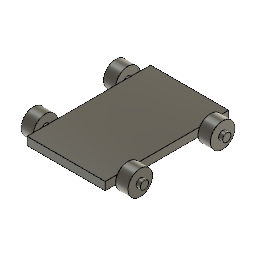
Semana3_DesafioExtra v1 (Autodesk Fusion 360 design; units mm, degrees)
Autodesk Fusion 360 part; units mm, degrees
sketch "Sketch2" plane through (0, 0, 0) normal (1, 0, 0) x (0, 1, 0)
  circle A0 centre (-50, 0) radius 15
  circle A1 centre (50, 0) radius 15
  dimension "d3" = 30
  dimension "d4" = 30
  dimension "d5" = 50
  dimension "d6" = 50
  constraint collinear origin A0.centre A1.centre
  measures "d3" diameter of A0
  measures "d4" diameter of A1
  measures "d5" distance of origin A0.centre
  measures "d6" distance of origin A1.centre
extrude "Extrude2" add sketch "Sketch2" along normal blind 15 makes body 1 at (10, 64.9255, -1.4935) makes body 2 at (10, -35.0745, -1.4935)
ref_plane "WorkPlane1" through (-100, 0, 0) normal (1, 0, 0) x (0, 1, 0)
sketch "Sketch3" plane through (-100, 0, 0) normal (1, 0, 0) x (0, 1, 0)
  circle A0 centre (50, 0) radius 15
  circle A1 centre (-50, 0) radius 15
  circle A2 centre (50, 0) radius 15
  circle A3 centre (-50, 0) radius 15
  dimension "d10" = 30
  dimension "d11" = 30
  constraint concentric A0 A2
  constraint concentric A1 A3
  measures "d10" diameter of A0
  measures "d11" diameter of A1
extrude "Extrude3" add sketch "Sketch3" against normal blind 15 separate body makes body 3 at (-110, 64.9255, -1.4935) makes body 4 at (-110, -35.0745, -1.4935)
sketch "Sketch4" plane through (15, 0, 0) normal (1, 0, 0) x (0, 1, 0)
  circle A0 centre (50, 0) radius 15
  circle A1 centre (50, 0) radius 5
  circle A2 centre (-50, 0) radius 5
  circle A3 centre (-50, 0) radius 15
  dimension "d14" = 10
  dimension "d15" = 10
  constraint concentric A0 A1
  constraint concentric A2 A3
  measures "d14" diameter of A1
  measures "d15" diameter of A2
extrude "Extrude4" add sketch "Sketch4" along normal blind -135 and the other way blind -5 contours A1 | A2 bodies 1 2 3 4
ref_plane "WorkPlane2" through (-52.6033, 50, 5) normal (0, 0, 1) x (0, -1, 0)
sketch "Sketch5" plane through (-52.6033, 50, 5) normal (0, 0, 1) x (1, 0, 0)
  line L0 (-45, -125) -> (50, -125)
  line L1 (50, -125) -> (50, 25)
  line L2 (50, 25) -> (-45, 25)
  line L3 (-45, 25) -> (-45, -125)
  dimension "d21" = 150
  constraint horizontal L0
  constraint perpendicular L0 L1
  constraint perpendicular L1 L2
  constraint perpendicular L0 L3
  measures "d21" distance of L0.start L2.end
extrude "Extrude5" add sketch "Sketch5" against normal blind 10 bodies 1 2
